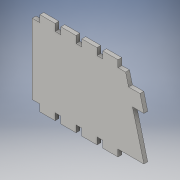
# Autodesk Inventor part: RTS Frame Sides
Saved by Autodesk Inventor 2016 (Build 200138000, 138)
## iProperties
Created: 2017-10-18
Part Number: RTS Frame Sides
Material: Generic
Document SubType Name: Modeling
Designer: student
Density: 1 g/cm^3
Appearance: Default
Author: student
Autodesk Inventor part; units mm, degrees
ref_plane "YZ Plane" through (0, 0, 0) normal (1, 0, 0) x (0, 1, 0)
ref_plane "XZ Plane" through (0, 0, 0) normal (0, 1, 0) x (-1, 0, 0)
ref_plane "XY Plane" through (0, 0, 0) normal (0, 0, 1) x (1, 0, 0)
sketch "Sketch1" plane through (0, 0, 0) normal (0, 0, 1) x (1, 0, 0)
  line L0 (-2.037, -23.495) -> (-2.037, -28.067)
  line L1 (-2.037, -28.067) -> (-12.197, -28.067)
  line L2 (-12.197, -28.067) -> (-12.197, -23.495)
  line L3 (-12.197, -23.495) -> (-16.007, -23.495)
  line L4 (-16.007, -23.495) -> (-16.007, -28.067)
  line L5 (-16.007, -28.067) -> (-26.167, -28.067)
  line L6 (-26.167, -28.067) -> (-26.167, -23.495)
  line L7 (-26.167, -23.495) -> (-29.977, -23.495)
  line L8 (-29.977, -23.495) -> (-29.977, -28.067)
  line L9 (-29.977, -28.067) -> (-40.137, -28.067)
  line L10 (-40.137, -28.067) -> (-40.137, -23.495)
  line L11 (-40.137, -23.495) -> (-43.947, -23.495)
  line L12 (-43.947, -23.495) -> (-43.947, -28.067)
  line L13 (-43.947, -28.067) -> (-54.107, -28.067)
  line L14 (-54.107, -28.067) -> (-54.107, -23.495)
  line L15 (-54.107, -23.495) -> (-59.187, -23.495)
  line L16 (3.043, 23.495) -> (-2.037, 23.495)
  line L17 (-2.037, 23.495) -> (-2.037, 28.067)
  line L18 (-2.037, 28.067) -> (-12.197, 28.067)
  line L19 (-12.197, 28.067) -> (-12.197, 23.495)
  line L20 (-12.197, 23.495) -> (-16.007, 23.495)
  line L21 (-16.007, 23.495) -> (-16.007, 28.067)
  line L22 (-16.007, 28.067) -> (-26.167, 28.067)
  line L23 (-26.167, 28.067) -> (-26.167, 23.495)
  line L24 (-26.167, 23.495) -> (-29.977, 23.495)
  line L25 (-29.977, 23.495) -> (-29.977, 28.067)
  line L26 (-29.977, 28.067) -> (-40.137, 28.067)
  line L27 (-40.137, 28.067) -> (-40.137, 23.495)
  line L28 (-40.137, 23.495) -> (-43.947, 23.495)
  line L29 (-43.947, 23.495) -> (-43.947, 28.067)
  line L30 (-43.947, 28.067) -> (-54.107, 28.067)
  line L31 (-54.107, 28.067) -> (-54.107, 23.495)
  line L32 (-54.107, 23.495) -> (-59.187, 23.495)
  line L33 (-59.187, 23.495) -> (-59.187, -23.495)
  line L34 (15.235, 5.7718) -> (15.235, 5.715)
  line L35 (15.235, 5.715) -> (7.6562, 5.715)
  line L36 (12.6136, 15.875) -> (15.235, 5.7718)
  line L37 (3.043, 23.495) -> (5.0201, 15.875)
  line L38 (7.6562, 5.715) -> (15.235, -23.495)
  line L39 (5.0201, 15.875) -> (12.6136, 15.875)
  line L40 (-2.037, -23.495) -> (15.235, -23.495)
  dimension "d11" = 4.572
  dimension "d12" = 10.16
  dimension "d13" = 3.81
  dimension "d14" = 10.16
  dimension "d15" = 3.81
  dimension "d16" = 10.16
  dimension "d17" = 3.81
  dimension "d18" = 10.16
  dimension "d19" = 5.08
  dimension "d34" = 4.572
  dimension "d84" = 7.62
  dimension "d85" = 29.21
  dimension "d86" = 10.1032
  constraints: 82 end point, 18 point on line, 12 perpendicular, 2 horizontal
  measures "d11" distance of L0.start L0.end
  measures "d12" distance of L0.end L1.end
  measures "d13" distance of L2.end L3.end
  measures "d14" distance of L4.end L5.end
  measures "d15" distance of L6.end L7.end
  measures "d16" distance of L8.end L9.end
  measures "d17" distance of L10.end L11.end
  measures "d18" distance of L12.end L13.end
  measures "d19" distance of L14.end L15.end
  measures "d34" distance of L11.end L12.end
  measures "d84" vertical distance of L16.start L37.end
  measures "d85" vertical distance of L35.end L38.end
  measures "d86" vertical distance of L36.start L34.start
extrude "Extrusion4" add sketch "Sketch1" along normal blind 2.54
body "Solid4"
